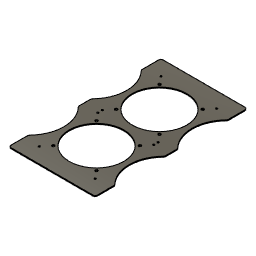
G5 Recessed Mount v3 (Autodesk Fusion 360 design; units mm, degrees)
Autodesk Fusion 360 part; units mm, degrees
sketch "Sketch1" plane through (0, 0, 0) normal (0, 0, 1) x (1, 0, 0)
  line L0 (3.175, 0) -> (122.301, 0)
  line L1 (125.476, -3.175) -> (125.476, -217.805)
  line L2 (122.301, -220.98) -> (3.175, -220.98)
  line L3 (0, -217.805) -> (0, -3.175)
  circle A0 centre (62.738, -64.77) radius 39.6875
  line L4 (94.1578, -33.3502) -> (31.3182, -33.3502) construction
  line L5 (31.3182, -33.3502) -> (31.3182, -96.1898) construction
  line L6 (31.3182, -96.1898) -> (94.1578, -96.1898) construction
  line L7 (94.1578, -96.1898) -> (94.1578, -33.3502) construction
  line L8 (94.1578, -33.3502) -> (31.3182, -96.1898) construction
  line L9 (31.3182, -33.3502) -> (94.1578, -96.1898) construction
  line L10 (103.251, -22.225) -> (22.225, -22.225) construction
  line L11 (22.225, -22.225) -> (22.225, -107.315) construction
  line L12 (22.225, -107.315) -> (103.251, -107.315) construction
  line L13 (103.251, -107.315) -> (103.251, -22.225) construction
  line L14 (103.251, -22.225) -> (22.225, -107.315) construction
  line L15 (22.225, -22.225) -> (103.251, -107.315) construction
  line L16 (62.738, -64.77) -> (62.738, 0) construction
  circle A1 centre (22.225, -22.225) radius 1.2446
  circle A2 centre (103.251, -22.225) radius 1.2446
  circle A3 centre (103.251, -107.315) radius 1.2446
  circle A4 centre (22.225, -107.315) radius 1.2446
  circle A5 centre (31.3182, -33.3502) radius 1.905
  circle A6 centre (94.1578, -33.3502) radius 1.905
  circle A7 centre (94.1578, -96.1898) radius 1.905
  circle A8 centre (31.3182, -96.1898) radius 1.905
  line L17 (0, -110.49) -> (125.476, -110.49) construction
  circle A9 centre (62.738, -156.21) radius 39.6875
  circle A10 centre (94.1578, -187.6298) radius 1.905
  circle A11 centre (103.251, -198.755) radius 1.2446
  circle A12 centre (31.3182, -187.6298) radius 1.905
  circle A13 centre (22.225, -198.755) radius 1.2446
  circle A14 centre (31.3182, -124.7902) radius 1.905
  circle A15 centre (22.225, -113.665) radius 1.2446
  circle A16 centre (94.1578, -124.7902) radius 1.905
  circle A17 centre (103.251, -113.665) radius 1.2446
  arc A18 (125.476, -3.175) -> (122.301, 0) centre (122.301, -3.175) ccw
  arc A19 (122.301, -220.98) -> (125.476, -217.805) centre (122.301, -217.805) ccw
  arc A20 (0, -217.805) -> (3.175, -220.98) centre (3.175, -217.805) ccw
  arc A21 (3.175, 0) -> (0, -3.175) centre (3.175, -3.175) ccw
  arc A22 (125.476, -28.4915) -> (125.476, -101.0485) centre (161.036, -64.77) ccw
  line L18 (106.426, 0) -> (106.426, -110.49) construction
  line L19 (110.236, -31.8716) -> (110.236, -89.3503) construction
  arc A23 (125.476, -119.9315) -> (125.476, -192.4885) centre (161.036, -156.21) ccw
  arc A24 (0, -101.0485) -> (0, -28.4915) centre (-35.56, -64.77) ccw
  arc A25 (0, -192.4885) -> (0, -119.9315) centre (-35.56, -156.21) ccw
  point P0 (125.476, 0)
  point P1 (0, -220.98)
  point P2 (62.738, -64.77)
  point P3 (62.738, -64.77)
  dimension "d1" = 125.476
  dimension "d2" = 220.98
  dimension "d5" = 64.77
  dimension "d8" = 22.225
  dimension "d9" = 33.3502
  dimension "d10" = 2.4892
  dimension "d11" = 3.81
  dimension "d12" = 96.1898
  dimension "d13" = 107.315
  dimension "d14" = 22.225
  dimension "d15" = 31.3182
  dimension "d16" = 94.1578
  dimension "d17" = 103.251
  dimension "d18" = 62.738
  dimension "d19" = 79.375
  dimension "d20" = 113.665
  dimension "d21" = 124.7902
  dimension "d22" = 156.21
  dimension "d23" = 187.6298
  dimension "d24" = 198.755
  dimension "d27" = 3.175
  dimension "d28" = 50.8
  dimension "d29" = 43.688
  dimension "d30" = 3.81
  constraint horizontal L0
  constraint vertical L1
  constraint horizontal L2
  constraint vertical L3
  constraint horizontal L4
  constraint perpendicular L4 L5
  constraint parallel L4 L6
  constraint parallel L5 L7
  constraint coincident L8 P3
  constraint coincident L9 P3
  constraint coincident P3 P2
  constraint horizontal L10
  constraint perpendicular L10 L11
  constraint parallel L10 L12
  constraint parallel L11 L13
  constraint coincident L14 P3
  constraint coincident L15 P3
  constraint equal L4 L7
  constraint vertical L16
  constraint coincident L10.end L11.start
  constraint coincident L10.start L13.end
  constraint coincident L12.end L13.start
  constraint coincident L11.end L12.start
  constraint equal A1 A2
  constraint equal A2 A3
  constraint equal A3 A4
  constraint coincident L4.end L5.start
  constraint coincident L4.start L7.end
  constraint coincident L6.end L7.start
  constraint coincident L5.end L6.start
  constraint equal A5 A6
  constraint equal A6 A7
  constraint equal A7 A8
  constraint symmetric A0 L17 A9
  constraint symmetric A1 L17 A13
  constraint symmetric A2 L17 A11
  constraint symmetric A3 L17 A17
  constraint symmetric A4 L17 A15
  constraint symmetric A5 L17 A12
  constraint symmetric A6 L17 A10
  constraint symmetric A7 L17 A16
  constraint symmetric A8 L17 A14
  constraint coincident L0 L16.end
  constraint coincident L1 L17.end
  constraint coincident P0 L0
  constraint coincident P0 L1
  constraint tangent L0 A18
  constraint tangent L1 A18
  constraint tangent L1 A19
  constraint tangent L2 A19
  constraint equal A18 A19
  constraint coincident L3 L17.start
  constraint coincident P1 L2
  constraint coincident P1 L3
  constraint tangent L2 A20
  constraint tangent L3 A20
  constraint equal A18 A20
  constraint coincident origin L3
  constraint coincident origin L0
  constraint tangent L3 A21
  constraint tangent L0 A21
  constraint equal A18 A21
  constraint midpoint L0 L16.end
  constraint midpoint L3 L17.start
  constraint midpoint L1 L17.end
  constraint coincident L1 A22.start
  constraint coincident L1 A22.end
  constraint horizontal P3 A22.centre
  constraint coincident L0 L18.start
  constraint coincident L17 L18.end
  constraint perpendicular L17 L18
  constraint tangent A22 L19
  constraint vertical L19
  constraint symmetric L17 A22.start A23.end
  constraint symmetric L17 A22.end A23.start
  constraint symmetric L17 A22 A23
  constraint symmetric L16 A22.start A24.end
  constraint symmetric L16 A22.end A24.start
  constraint symmetric L16 A22 A24
  constraint symmetric L16 A23.end A25.start
  constraint symmetric L16 A23.start A25.end
  constraint symmetric L16 A23 A25
  measures "d1" distance of origin P0
  measures "d2" distance of origin P1
  measures "d5" distance of L0 P3
  measures "d8" distance of L0 L10
  measures "d9" distance of L0 L4
  measures "d10" diameter of A1
  measures "d11" diameter of A5
  measures "d12" distance of L0 L5.end
  measures "d13" distance of L0 L11.end
  measures "d14" distance of L3 L10.end
  measures "d15" distance of L3 L4.end
  measures "d16" distance of L3 L4.start
  measures "d17" distance of L3 L13
  measures "d18" distance of L3 L16
  measures "d19" diameter of A0
  measures "d20" distance of L0 A15.centre
  measures "d21" distance of L0 A14.centre
  measures "d22" distance of L0 A9.centre
  measures "d23" distance of L0 A12.centre
  measures "d24" distance of L0 A13.centre
  measures "d27" radius of A18
  measures "d28" radius of A22
  measures "d29" distance of P3 L18
  measures "d30" distance of L18 L19
extrude "Extrude1" add sketch "Sketch1" along normal blind 1.27 contours L0 L1 L2 L3 A18 A19 A20 A21 A22 A23 A24 A25
fillet "Fillet1" radius 3.175 8 edges at (125.476, -28.4915, 0.635) (125.476, -101.0485, 0.635) (125.476, -119.9315, 0.635) (125.476, -192.4885, 0.635) (0, -192.4885, 0.635) (0, -119.9315, 0.635) (0, -101.0485, 0.635) (0, -28.4915, 0.635)
equation "d29 = ( 3.44 / 2 ) * 1 in"
